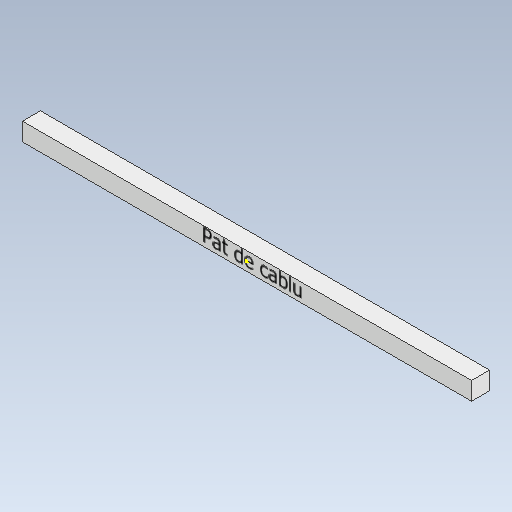
# Autodesk Inventor part: 0005-10-1017 pat de cablu
Saved by Autodesk Inventor 2020 (Build 240168000, 168)
## iProperties
Created: 2020-12-19
Part Number: 0005-10-1017 pat de cablu
Material: Generic
Document SubType Name: Modeling
Designer: Iulian Bors
Density: 1 g/cm^3
Appearance: Default(1)
Author: Iulian Bors
Subject: 20-1017
Autodesk Inventor part; units mm, degrees
ref_plane "YZ Plane" through (0, 0, 0) normal (1, 0, 0) x (0, 1, 0)
ref_plane "XZ Plane" through (0, 0, 0) normal (0, 1, 0) x (-1, 0, 0)
ref_plane "XY Plane" through (0, 0, 0) normal (0, 0, 1) x (1, 0, 0)
sketch "Sketch1" plane through (0, 0, 0) normal (0, 0, 1) x (1, 0, 0)
  line L0 (-250, 10) -> (250, 10)
  line L1 (250, 10) -> (250, -10)
  line L2 (250, -10) -> (-250, -10)
  line L3 (-250, -10) -> (-250, 10)
  point P0 (0, 0)
  point P1 (-250, 0)
  point P2 (0, 10)
  dimension "d0" = 20
  dimension "d1" = 500
  constraints: 8 end point, 2 midpoint, 2 parallel, 1 horizontal, 1 horizontal alignment, 1 perpendicular, 1 vertical alignment
  measures "d0" distance of L2.end L0.start
  measures "d1" distance of L0.start L0.end
extrude "Extrusion1" add sketch "Sketch1" along normal blind 20
sketch "Sketch2" plane through (0, 0, 20) normal (0, 0, 1) x (1, 0, 0)
  line L0 (-50.1977, 9.8362) -> (224.6394, 9.8362) construction
  line L1 (224.6394, 9.8362) -> (224.6394, 2.2903) construction
  line L2 (224.6394, 2.2903) -> (-50.1977, 2.2903) construction
  line L3 (-50.1977, 2.2903) -> (-50.1977, 9.8362) construction
  point P0 (0, 0)
  constraints: 2 other
body "Solid1"
